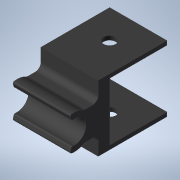
# Autodesk Inventor part: Stengelihalter
Saved by Autodesk Inventor 2021 (Build 250183000, 183)
## iProperties
Created: 2024-02-11
Part Number: Stengelihalter
Material: Generic
Document SubType Name: Modeling
Designer: Lukas
Density: 1 g/cm^3
Appearance: Default
Author: Lukas
Autodesk Inventor part; units mm, degrees
ref_plane "YZ Plane" through (0, 0, 0) normal (1, 0, 0) x (0, 1, 0)
ref_plane "XZ Plane" through (0, 0, 0) normal (0, 1, 0) x (-1, 0, 0)
ref_plane "XY Plane" through (0, 0, 0) normal (0, 0, 1) x (1, 0, 0)
sketch "Sketch1" plane through (0, 0, 0) normal (0, 0, 1) x (1, 0, 0)
  line L0 (-10, 11.5) -> (10, 11.5)
  line L1 (10, 11.5) -> (10, -11.5)
  line L2 (10, -11.5) -> (-10, -11.5)
  line L3 (-10, -11.5) -> (-10, 11.5)
  point P0 (0, 0)
  point P1 (0, 11.5)
  point P2 (-10, 0)
  dimension "d0" = 20
  dimension "d16" = 23
  constraints: 8 end point, 2 midpoint, 2 parallel, 1 horizontal, 1 horizontal alignment, 1 perpendicular, 1 vertical alignment
  measures "d0" distance of L0.start L0.end
  measures "d16" distance of L2.end L0.start
extrude "Extrusion1" add sketch "Sketch1" along normal blind 4
sketch "Sketch2" plane through (0, 0, 0) normal (1, 0, 0) x (0, 1, 0)
  line L0 (11.5, 0) -> (-11.5, 0) projected
  line L1 (-11.5, 0) -> (-11.5, 4) projected
  line L2 (11.5, 4) -> (-11.5, 4) projected
  line L3 (11.5, 0) -> (11.5, 4) projected
  line L4 (5, 4) -> (5, 9)
  line L5 (-5, 4) -> (-5, 9)
  arc A0 (-5.7956, 13.8695) -> (5.7956, 13.8695) centre (0, 12.3166) ccw
  arc A1 (-3.8637, 13.3519) -> (3.8637, 13.3519) centre (0, 12.3166) ccw
  line L6 (3.8637, 13.3519) -> (5.7956, 13.8695)
  line L7 (-5.7956, 13.8695) -> (-3.8637, 13.3519)
  point P0 (0, 0)
  point P1 (0, 0)
  dimension "d3" = 6
  dimension "d4" = 5
  dimension "d5" = 4
  dimension "d6" = 10
  dimension "d8" = 150
  constraints: 8 end point, 6 point on circle, 2 centre point, 2 line through centre, 2 perpendicular, 2 point on line, 1 coincident, 1 horizontal alignment, 1 midpoint, 1 parallel, 1 vertical alignment
  measures "d3" radius of A0
  measures "d4" distance of L4.start L4.end
  measures "d5" radius of A1
  measures "d6" distance between parallel lines of L5 L4
  measures "d8" angle of L7 L6
extrude "Extrusion2" add sketch "Sketch2" along normal mid plane 20 contours L2 L5 A0 L4 | A0 L7 A1 L6
fillet "Fillet1" radius 2 4 edges at (0, -5, 4) (0, -5, 9) (0, 5, 9) (0, 5, 4)
fillet "Fillet2" radius 0.5 4 edges at (0, 3.8637, 13.3519) (0, 5.7956, 13.8695) (0, -3.8637, 13.3519) (0, -5.7956, 13.8695)
sketch "Sketch4" plane through (0, 0, 0) normal (0, 0, -1) x (-1, 0, 0)
  line L0 (-10, -11.5) -> (-10, 11.5) projected
  line L1 (10, 11.5) -> (10, -11.5) projected
  line L2 (-10, 11.5) -> (10, 11.5)
  line L3 (10, 11.5) -> (10, 10.1)
  line L4 (10, 10.1) -> (-10, 10.1)
  line L5 (-10, 10.1) -> (-10, 11.5)
  line L6 (10, -11.5) -> (-10, -11.5) projected
  line L7 (-10, -11.5) -> (10, -11.5)
  line L8 (10, -11.5) -> (10, -10.1)
  line L9 (10, -10.1) -> (-10, -10.1)
  line L10 (-10, -10.1) -> (-10, -11.5)
  point P0 (0, 0)
  point P1 (-10, -10.1)
  point P2 (-10, 10.1)
  dimension "d17" = 1.4
  constraints: 16 end point, 4 parallel, 2 horizontal, 2 perpendicular, 2 point on line, 1 collinear
  measures "d17" distance of L2.end L3.end
extrude "Extrusion3" add sketch "Sketch4" along normal blind 20 contours L0 L9 L1 L6 | L0 L2 L1 L4
sketch "Sketch5" plane through (-10, -11.5, 4) normal (0, -1, 0) x (1, 0, 0)
  line L0 (0, -4) -> (20, -4) projected
  line L1 (0, -4) -> (0, -24) projected
  line L2 (20, -24) -> (0, -24) projected
  line L3 (20, -4) -> (20, -24) projected
  circle A0 centre (10, -14) radius 2.15
  point P0 (10, -4)
  point P1 (0, -14)
  dimension "d20" = 4.3
  constraints: 1 centre point, 1 horizontal alignment, 1 midpoint, 1 vertical alignment
  measures "d20" diameter of A0
extrude "Extrusion4" cut sketch "Sketch5" against normal through all contours A0
body "Solid1"
